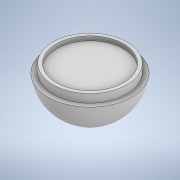
# Autodesk Inventor part: bottom ball bottom
Saved by Autodesk Inventor 2022 (Build 260153000, 153)
## iProperties
Created: 2022-03-14
Part Number: bottom ball bottom
Material: Generic
Document SubType Name: Modeling
Designer: mogje
Density: 1 g/cm^3
Appearance: Default
Author: mogje
Autodesk Inventor part; units mm, degrees
ref_plane "YZ Plane" through (0, 0, 0) normal (1, 0, 0) x (0, 1, 0)
ref_plane "XZ Plane" through (0, 0, 0) normal (0, 1, 0) x (-1, 0, 0)
ref_plane "XY Plane" through (0, 0, 0) normal (0, 0, 1) x (1, 0, 0)
sketch "Sketch1" plane through (0, 0, 0) normal (0, 1, 0) x (-1, 0, 0)
  arc A0 (31.75, 0) -> (-31.75, 0) centre (0, 0) ccw
  line L0 (0, 0) -> (-31.75, 0) construction
  line L1 (0, 0) -> (31.75, 0) construction
  line L2 (31.75, 0) -> (-31.75, 0)
  dimension "d0" = 31.75
  dimension "d1" = 180
  constraints: 6 end point, 4 point on circle, 1 centre point, 1 coincident
  measures "d0" radius of A0
  measures "d1" angle of L0 L1
revolve "Revolution1" add sketch "Sketch1" angle 180 about axis through (-31.75, 0, 0) along (1, 0, 0)
sketch "Sketch2" plane through (0, 0, 0) normal (0, 1, 0) x (1, 0, 0)
  line L0 (0, 0) -> (0, 27.94)
  line L1 (0, 0) -> (0, 25.4)
  circle A0 centre (0, 0) radius 27.94
  circle A1 centre (0, 0) radius 25.4
  dimension "d3" = 27.94
  dimension "d4" = 25.4
  constraints: 4 end point, 2 coincident, 2 vertical alignment, 1 point on line, 1 vertical, 4 other
  measures "d3" distance of L0.start L0.end
  measures "d4" distance of L0.start L1.end
extrude "Extrusion1" add sketch "Sketch2" along normal blind 3.175
sketch "Sketch3" plane through (0, 0, 0) normal (0, 1, 0) x (1, 0, 0)
  circle A0 centre (0, 0) radius 27.94
  circle A1 centre (0, 0) radius 31.75
  constraints: 2 centre point, 2 coincident
extrude "Extrusion2" cut sketch "Sketch3" against normal blind 3.175
body "Solid1"
